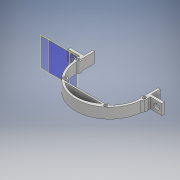
# Autodesk Inventor part: anneaustop
Saved by Autodesk Inventor 2017 (Build 210142000, 142)
## iProperties
Part Number: anneaustop
Material: Générique
Document SubType Name: Modeling
Designer: Thomas
Density: 1 g/cm^3
Appearance: Par défaut
Author: Thomas
Autodesk Inventor part; units mm, degrees
ref_plane "YZ Plane" through (0, 0, 0) normal (1, 0, 0) x (0, 1, 0)
ref_plane "XZ Plane" through (0, 0, 0) normal (0, 1, 0) x (-1, 0, 0)
ref_plane "XY Plane" through (0, 0, 0) normal (0, 0, 1) x (1, 0, 0)
sketch "Esquisse1" plane through (0, 0, 0) normal (0, 0, 1) x (1, 0, 0)
  line L0 (0, 0) -> (-27.546, -25.0426) construction
  line L1 (0, 0) -> (23.0277, -27.4577) construction
  circle A0 centre (-18.0975, -16.4528) radius 1.25
  circle A1 centre (15.7127, -18.7355) radius 1.25
  arc A2 (-16.6894, -17.8731) -> (14.1299, -19.9581) centre (0, 0) ccw
  arc A3 (-16.6894, -17.8731) -> (-19.3824, -14.9201) centre (-18.0975, -16.4528) ccw
  arc A4 (17.0433, -17.2424) -> (14.1299, -19.9581) centre (15.7127, -18.7355) ccw
  line L2 (0, 0) -> (-29.5508, 10.7556) construction
  line L3 (-17.8311, 0) -> (17.1748, 0) construction
  line L4 (0, 2.0526) -> (0, -2.2236) construction
  arc A5 (-25.923, -2) -> (25.923, -2) centre (0, 0) ccw
  circle A6 centre (0, 0) radius 22.5 construction
  arc A7 (-16.6894, -17.8731) -> (14.1299, -19.9581) centre (0, 0) ccw
  arc A8 (-16.6894, -17.8731) -> (14.1299, -19.9581) centre (0, 0) ccw
  circle A9 centre (-25.3169, 1.1605) radius 1.25
  circle A10 centre (25.3169, 1.1605) radius 1.25
  line L5 (24.0891, 2.7784) -> (24.0891, 12.8348)
  line L6 (25.8363, 12.8348) -> (24.0891, 12.8348)
  line L7 (-25.923, 6.143) -> (-25.923, 12.7847)
  line L8 (-24.2942, 2.9148) -> (-24.2942, 12.7847)
  line L9 (-24.2942, 12.7847) -> (-25.923, 12.7847)
  arc A11 (-24.4506, -0.676) -> (-19.3824, -14.9201) centre (0, 0) ccw
  arc A12 (-24.4506, -0.676) -> (-19.3824, -14.9201) centre (0, 0) ccw
  arc A13 (-24.4506, -0.676) -> (-24.2942, 2.9148) centre (-25.3169, 1.1605) ccw
  arc A14 (17.0433, -17.2424) -> (24.2376, -0.5599) centre (0, 0) ccw
  arc A15 (17.0433, -17.2424) -> (24.2376, -0.5599) centre (0, 0) ccw
  arc A16 (17.0433, -17.2424) -> (24.2376, -0.5599) centre (0, 0) ccw
  arc A17 (24.0891, 2.7784) -> (24.2376, -0.5599) centre (25.3169, 1.1605) ccw
  line L10 (25.8363, 3.0919) -> (25.8363, 3.124)
  line L11 (25.8363, 6.3239) -> (25.8363, 12.8348)
  line L12 (25.8363, 6.3239) -> (25.9915, 6)
  line L13 (-36, 4) -> (-26.9495, 4)
  line L14 (-36, 6) -> (-26, 6)
  line L15 (-36, 4) -> (-36, 6)
  line L16 (-26, 6) -> (-25.9915, 6)
  line L17 (-25.9915, 6) -> (-25.923, 6.143)
  line L18 (-26.9495, 4) -> (-26.9495, 2.3678)
  line L19 (-25.923, -2) -> (-26.9495, -0.0468)
  arc A18 (-26.9495, 2.3678) -> (-26.9495, -0.0468) centre (-25.3169, 1.1605) ccw
  arc A19 (-24.4506, -0.676) -> (-24.2942, 2.9148) centre (-25.3169, 1.1605) ccw
  line L20 (25.9915, 6) -> (25.923, 6.143)
  line L21 (36, 4) -> (26.9495, 4)
  line L22 (36, 6) -> (26, 6)
  line L23 (36, 4) -> (36, 6)
  line L24 (26.9495, 4) -> (26.9495, 2.3678)
  line L25 (25.923, -2) -> (26.9495, -0.0468)
  arc A20 (26.9495, -0.0468) -> (26.9495, 2.3678) centre (25.3169, 1.1605) ccw
  line L26 (25.9915, 6) -> (26, 6)
  point P0 (29.8237, -2)
  point P1 (-36, -2)
  point P2 (-26.3114, 9.5766)
  dimension "d35" = 2.5
  dimension "d36" = 2.5
  dimension "d37" = 4
  dimension "d38" = 4
  dimension "d39" = 20
  dimension "d52" = 45
  dimension "d65" = 2.5
  dimension "d81" = 10
  constraints: 54 end point, 33 point on circle, 21 centre point, 10 symmetric about line, 8 coincident, 8 vertical, 7 point on line, 5 horizontal, 2 perpendicular, 2 other
  measures "d35" diameter of A0
  measures "d36" diameter of A1
  measures "d37" diameter of A3
  measures "d38" diameter of A4
  measures "d39" angle of L3 L2
  measures "d52" diameter of A6
  measures "d65" diameter of A9
  measures "d81" distance of L14.start L14.end
ref_plane "Plan de construction1" through (-42, 0, 0) normal (0, 1, 0) x (1, 0, 0)
ref_plane "Plan de construction2" through (-36, 0, 0) normal (0, 1, 0) x (1, 0, 0)
sketch "Esquisse3" plane through (-36, 0, 0) normal (0, 1, 0) x (1, 0, 0)
  line L0 (0, 0) -> (10, 0) projected
  line L1 (0, 0) -> (0, -8) projected
  line L2 (10, -8) -> (0, -8) projected
  line L3 (10, 0) -> (10, -8) projected
  circle A0 centre (4, -4) radius 2.15
  line L4 (62, 0) -> (72, 0) projected
  line L5 (62, 0) -> (62, -8) projected
  line L6 (72, -8) -> (62, -8) projected
  line L7 (72, 0) -> (72, -8) projected
  circle A1 centre (68, -4) radius 2.15
  point P0 (36, 0)
  dimension "d48" = 4.3
  dimension "d73" = 4
  dimension "d74" = 4.3
  dimension "d75" = 4
  constraints: 2 centre point
  measures "d48" diameter of A0
  measures "d73" distance from line of L1 A0.centre
  measures "d74" diameter of A1
  measures "d75" distance from line of L7 A1.centre
extrude "Extrusion16" add sketch "Esquisse1" along normal blind 8
extrude "Extrusion17" cut sketch "Esquisse3" along normal blind 8 contours A0 | A1
sketch "Esquisse5" plane through (0, 0, 8) normal (0, 0, 1) x (1, 0, 0)
  arc A0 (-16.6894, -17.8731) -> (14.1299, -19.9581) centre (0, 0) ccw projected
  circle A1 centre (25.3169, 1.1605) radius 1.25 projected
  circle A2 centre (-25.3169, 1.1605) radius 1.25 projected
  circle A3 centre (15.7127, -18.7355) radius 1.25 projected
  circle A4 centre (-18.0975, -16.4528) radius 1.25 projected
  arc A5 (-16.6894, -17.8731) -> (-19.3824, -14.9201) centre (-18.0975, -16.4528) ccw projected
  arc A6 (-24.4506, -0.676) -> (-19.3824, -14.9201) centre (0, 0) ccw projected
  arc A7 (-24.4506, -0.676) -> (-24.2942, 2.9148) centre (-25.3169, 1.1605) ccw projected
  line L0 (-24.2942, 2.9148) -> (-24.2942, 12.7847) projected
  line L1 (-24.2942, 12.7847) -> (-25.923, 12.7847) projected
  line L2 (-25.923, 12.7847) -> (-25.923, 6.143) projected
  line L3 (-25.923, 6.143) -> (-25.9915, 6) projected
  line L4 (-25.9915, 6) -> (-36, 6) projected
  line L5 (-36, 6) -> (-36, 4) projected
  line L6 (-36, 4) -> (-26.9495, 4) projected
  line L7 (-26.9495, 4) -> (-26.9495, 2.3678) projected
  arc A8 (-26.9495, 2.3678) -> (-26.9495, -0.0468) centre (-25.3169, 1.1605) ccw projected
  line L8 (-26.9495, -0.0468) -> (-25.923, -2) projected
  arc A9 (-25.923, -2) -> (25.923, -2) centre (0, 0) ccw projected
  line L9 (25.923, -2) -> (26.9495, -0.0468) projected
  arc A10 (26.9495, -0.0468) -> (26.9495, 2.3678) centre (25.3169, 1.1605) ccw projected
  line L10 (26.9495, 2.3678) -> (26.9495, 4) projected
  line L11 (26.9495, 4) -> (36, 4) projected
  line L12 (36, 4) -> (36, 6) projected
  line L13 (36, 6) -> (25.9915, 6) projected
  line L14 (25.9915, 6) -> (25.8363, 6.3239) projected
  line L15 (25.8363, 6.3239) -> (25.8363, 12.8348) projected
  line L16 (25.8363, 12.8348) -> (24.0891, 12.8348) projected
  line L17 (24.0891, 12.8348) -> (24.0891, 2.7784) projected
  arc A11 (24.0891, 2.7784) -> (24.2376, -0.5599) centre (25.3169, 1.1605) ccw projected
  arc A12 (17.0433, -17.2424) -> (24.2376, -0.5599) centre (0, 0) ccw projected
  arc A13 (17.0433, -17.2424) -> (14.1299, -19.9581) centre (15.7127, -18.7355) ccw projected
  arc A14 (-16.6894, -17.8731) -> (14.1299, -19.9581) centre (0, 0) ccw projected
  line L18 (-16.356, -17.8956) -> (-16.6894, -17.8731)
  arc A15 (17.0433, -17.2424) -> (14.1299, -19.9581) centre (15.7127, -18.7355) ccw projected
  arc A16 (13.8936, -17.9043) -> (-16.356, -17.8956) centre (-8.178, -24366.3326) ccw
  arc A17 (-16.6894, -17.8731) -> (-19.3824, -14.9201) centre (-18.0975, -16.4528) ccw projected
  arc A18 (-16.6894, -17.8731) -> (14.1299, -19.9581) centre (0, 0) ccw
  arc A19 (13.8936, -17.9043) -> (14.1299, -19.9581) centre (15.7127, -18.7355) ccw
  constraints: 9 point on circle, 3 centre point, 2 end point
extrude "Extrusion18" add sketch "Esquisse5" against normal blind 8 contours L18 A16 A13 A0
sketch "Esquisse6" plane through (0, 0, 8) normal (0, 0, 1) x (1, 0, 0)
  circle A0 centre (25.3169, 1.1605) radius 1.25 projected
  circle A1 centre (-25.3169, 1.1605) radius 1.25 projected
  circle A2 centre (15.7127, -18.7355) radius 1.25 projected
  circle A3 centre (-18.0975, -16.4528) radius 1.25 projected
  arc A4 (-16.6894, -17.8731) -> (-19.3824, -14.9201) centre (-18.0975, -16.4528) ccw projected
  arc A5 (-24.4506, -0.676) -> (-19.3824, -14.9201) centre (0, 0) ccw projected
  arc A6 (-24.4506, -0.676) -> (-24.2942, 2.9148) centre (-25.3169, 1.1605) ccw projected
  line L0 (-24.2942, 2.9148) -> (-24.2942, 12.7847) projected
  line L1 (-24.2942, 12.7847) -> (-25.923, 12.7847) projected
  line L2 (-25.923, 12.7847) -> (-25.923, 6.143) projected
  line L3 (-25.923, 6.143) -> (-25.9915, 6) projected
  line L4 (-25.9915, 6) -> (-36, 6) projected
  line L5 (-36, 6) -> (-36, 4) projected
  line L6 (-36, 4) -> (-26.9495, 4) projected
  line L7 (-26.9495, 4) -> (-26.9495, 2.3678) projected
  arc A7 (-26.9495, 2.3678) -> (-26.9495, -0.0468) centre (-25.3169, 1.1605) ccw projected
  line L8 (-26.9495, -0.0468) -> (-25.923, -2) projected
  arc A8 (-25.923, -2) -> (25.923, -2) centre (0, 0) ccw projected
  line L9 (25.923, -2) -> (26.9495, -0.0468) projected
  arc A9 (26.9495, -0.0468) -> (26.9495, 2.3678) centre (25.3169, 1.1605) ccw projected
  line L10 (26.9495, 2.3678) -> (26.9495, 4) projected
  line L11 (26.9495, 4) -> (36, 4) projected
  line L12 (36, 4) -> (36, 6) projected
  line L13 (36, 6) -> (25.9915, 6) projected
  line L14 (25.9915, 6) -> (25.8363, 6.3239) projected
  line L15 (25.8363, 6.3239) -> (25.8363, 12.8348) projected
  line L16 (25.8363, 12.8348) -> (24.0891, 12.8348) projected
  line L17 (24.0891, 12.8348) -> (24.0891, 2.7784) projected
  arc A10 (24.0891, 2.7784) -> (24.2376, -0.5599) centre (25.3169, 1.1605) ccw projected
  arc A11 (17.0433, -17.2424) -> (24.2376, -0.5599) centre (0, 0) ccw projected
  arc A12 (17.0433, -17.2424) -> (13.8936, -17.9043) centre (15.7127, -18.7355) ccw projected
  arc A13 (13.8936, -17.9043) -> (-16.356, -17.8956) centre (-8.178, -24366.3326) ccw projected
  line L18 (-16.356, -17.8956) -> (-16.6894, -17.8731) projected
  line L19 (-15.3155, -19.0715) -> (12.9977, -19.0715)
  arc A14 (-15.3155, -19.0715) -> (12.9977, -19.0715) centre (-1.1589, -2.415) ccw
  constraints: 2 end point, 2 point on circle, 1 centre point, 1 horizontal
extrude "Extrusion19" cut sketch "Esquisse6" against normal blind 8 contours L19 A14
